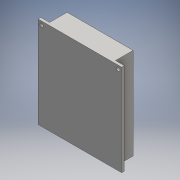
# Autodesk Inventor part: CPD Module
Saved by Autodesk Inventor 2016 (Build 200138000, 138)
## iProperties
Created: 2016-01-08
Part Number: CPD Module
Material: Generic
Document SubType Name: Modeling
Designer: TimB
Density: 1 g/cm^3
Appearance: Default
Author: TimB
Autodesk Inventor part; units mm, degrees
ref_plane "YZ Plane" through (0, 0, 0) normal (1, 0, 0) x (0, 1, 0)
ref_plane "XZ Plane" through (0, 0, 0) normal (0, 1, 0) x (-1, 0, 0)
ref_plane "XY Plane" through (0, 0, 0) normal (0, 0, 1) x (1, 0, 0)
sketch "Sketch1" plane through (0, 0, 0) normal (0, 1, 0) x (-1, 0, 0)
  line L0 (-47.5, -52) -> (47.5, -52)
  line L1 (47.5, -52) -> (47.5, 52)
  line L2 (47.5, 52) -> (-47.5, 52)
  line L3 (-47.5, 52) -> (-47.5, -52)
  line L4 (-47.5, -52) -> (47.5, 52) construction
  line L5 (47.5, -52) -> (-47.5, 52) construction
  point P0 (0, 0)
  dimension "d0" = 95
  dimension "d1" = 104
  constraints: 12 end point, 2 midpoint, 2 parallel, 1 horizontal, 1 perpendicular
  measures "d0" distance of L2.end L1.end
  measures "d1" distance of L1.end L0.end
extrude "Extrusion1" add sketch "Sketch1" along normal blind 3
sketch "Sketch2" plane through (0, 3, 0) normal (0, 1, 0) x (1, 0, 0)
  line L0 (-47.5, -52) -> (47.5, -52) projected
  line L1 (37.5, 52) -> (-37.5, 52)
  line L2 (-37.5, 52) -> (-37.5, -52)
  line L3 (-37.5, -52) -> (37.5, -52)
  line L4 (37.5, -52) -> (37.5, 52)
  line L5 (37.5, 52) -> (-37.5, -52) construction
  line L6 (-37.5, 52) -> (37.5, -52) construction
  point P0 (0, 0)
  dimension "d4" = 75
  dimension "d5" = 104
  constraints: 12 end point, 2 midpoint, 2 parallel, 1 horizontal, 1 perpendicular, 1 point on line
  measures "d4" distance of L3.end L2.end
  measures "d5" distance of L1.end L2.end
extrude "Extrusion2" add sketch "Sketch2" along normal blind 20
sketch "Sketch3" plane through (0, 0, 0) normal (0, -1, 0) x (1, 0, 0)
  line L0 (-47.5, 52) -> (-43.5, 52)
  line L1 (-43.5, 52) -> (-43.5, 48)
  line L2 (-43.5, 48) -> (-47.5, 48)
  line L3 (-47.5, 48) -> (-47.5, 52)
  line L4 (-47.5, 52) -> (47.5, 52) projected
  line L5 (47.5, 52) -> (43.5, 52)
  line L6 (43.5, 52) -> (43.5, 48)
  line L7 (43.5, 48) -> (47.5, 48)
  line L8 (47.5, 48) -> (47.5, 52)
  point P0 (0, 0)
  dimension "d8" = 4
  dimension "d9" = 4
  dimension "d10" = 4
  dimension "d11" = 4
  constraints: 16 end point, 4 parallel, 2 horizontal, 2 perpendicular
  measures "d8" distance of L1.end L2.end
  measures "d9" distance of L0.end L1.end
  measures "d10" distance of L7.end L6.end
  measures "d11" distance of L6.end L5.end
hole "Hole1" at (-43.5, 0, 48) at (43.5, 0, 48) direction (0, 1, 0) diameter 4 end through all
body "Solid1"
